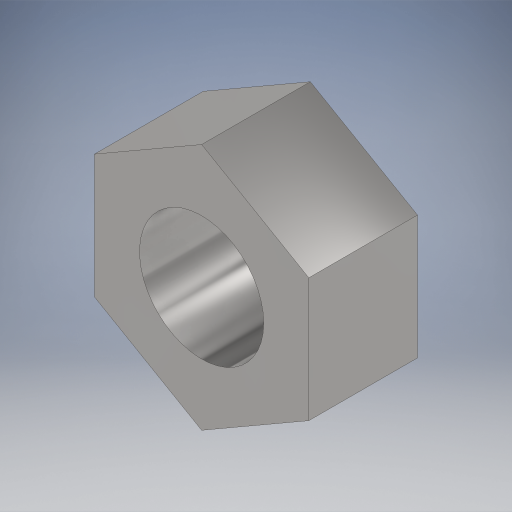
# Autodesk Inventor part: Болт м4
Saved by Autodesk Inventor 2023 (Build 270158000, 158)
## iProperties
Created: 2023-01-05
Part Number: Болт м4
Material: Типовые
Document SubType Name: Modeling
Designer: Admin
Density: 1 g/cm^3
Appearance: По умолчанию
Author: Admin
Autodesk Inventor part; units mm, degrees
ref_plane "YZ Plane" through (0, 0, 0) normal (1, 0, 0) x (0, 1, 0)
ref_plane "XZ Plane" through (0, 0, 0) normal (0, 1, 0) x (-1, 0, 0)
ref_plane "XY Plane" through (0, 0, 0) normal (0, 0, 1) x (1, 0, 0)
sketch "Эскиз1" plane through (0, 0, 0) normal (0, 0, 1) x (1, 0, 0)
  line L0 (3.45, 1.9919) -> (3.45, -1.9919)
  line L1 (3.45, -1.9919) -> (0, -3.9837)
  line L2 (0, -3.9837) -> (-3.45, -1.9919)
  line L3 (-3.45, -1.9919) -> (-3.45, 1.9919)
  line L4 (-3.45, 1.9919) -> (0, 3.9837)
  line L5 (0, 3.9837) -> (3.45, 1.9919)
  circle A0 centre (0, 0) radius 2
  dimension "d0" = 6.9
  dimension "d1" = 4
  constraints: 12 end point, 2 coincident, 1 centre point, 1 vertical, 13 other
  measures "d0" distance between parallel lines of L3 L0
  measures "d1" diameter of A0
extrude "Выдавливание1" add sketch "Эскиз1" along normal blind 3.5
